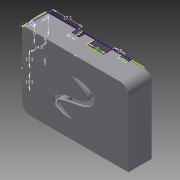
# Autodesk Inventor part: bottom
Saved by Autodesk Inventor 2015 (Build 190159000, 159)
## iProperties
Created: 2015-01-18
Part Number: bottom
Material: Generic
Document SubType Name: Modeling
Designer: Bardo91
Density: 1 g/cm^3
Appearance: Default
Author: Bardo91
Autodesk Inventor part; units mm, degrees
ref_plane "YZ Plane" through (0, 0, 0) normal (1, 0, 0) x (0, 1, 0)
ref_plane "XZ Plane" through (0, 0, 0) normal (0, 1, 0) x (-1, 0, 0)
ref_plane "XY Plane" through (0, 0, 0) normal (0, 0, 1) x (1, 0, 0)
sketch "baseBody" plane through (0, 0, 0) normal (0, 1, 0) x (-1, 0, 0)
  line L0 (50, 35) -> (-42, 35)
  line L1 (-50, 27) -> (-50, -35)
  line L2 (-50, -35) -> (42, -35)
  line L3 (50, -27) -> (50, 35)
  arc A0 (42, -35) -> (50, -27) centre (42, -27) ccw
  arc A1 (-42, 35) -> (-50, 27) centre (-42, 27) ccw
  point P0 (-50, 35)
  point P1 (50, -35)
  point P2 (0, 0)
  dimension "d175" = 100
  dimension "d176" = 70
  dimension "d177" = 50
  dimension "d178" = 35
  dimension "d179" = 8
  constraints: 8 end point, 4 point on circle, 4 point on line, 4 tangent, 2 centre point, 2 parallel, 1 equal radius, 1 horizontal, 1 perpendicular
  measures "d175" distance of point (50, -35) L1.end
  measures "d176" distance of point (-50, 35) L1.end
  measures "d177" distance from line of L1 point (0, 0)
  measures "d178" distance from line of L0 point (0, 0)
  measures "d179" radius of A0
extrude "Body" add sketch "baseBody" along normal blind 23
shell "case" thickness 2 removed faces 1 at (-16.6667, 23, 11.6667)
sketch "baseBorder" plane through (0, 23, 0) normal (0, 1, 0) x (1, 0, 0)
  line L0 (-50, -35) -> (42, -35)
  line L1 (50, -27) -> (50, 35)
  line L2 (50, 35) -> (-42, 35)
  line L3 (-50, 27) -> (-50, -35)
  arc A0 (-42, 35) -> (-50, 27) centre (-42, 27) ccw
  arc A1 (42, -35) -> (50, -27) centre (42, -27) ccw
  line L4 (42, -34) -> (-49, -34)
  line L5 (-49, -34) -> (-49, 27)
  arc A2 (-42, 34) -> (-49, 27) centre (-42, 27) ccw
  line L6 (-42, 34) -> (49, 34)
  line L7 (49, 34) -> (49, -27)
  arc A3 (42, -34) -> (49, -27) centre (42, -27) ccw
  line L8 (-48, -33) -> (42, -33)
  arc A4 (42, -33) -> (48, -27) centre (42, -27) ccw
  line L9 (48, -27) -> (48, 33)
  line L10 (48, 33) -> (-42, 33)
  arc A5 (-42, 33) -> (-48, 27) centre (-42, 27) ccw
  line L11 (-48, 27) -> (-48, -33)
  point P0 (0, 0)
  dimension "d181" = 8
  dimension "d182" = 1
  dimension "d183" = 1
  constraints: 24 end point, 12 point on circle, 6 centre point, 6 parallel, 4 tangent, 3 perpendicular, 1 equal radius, 1 horizontal, 10 other
  measures "d181" radius of A0
  measures "d182" distance between parallel lines of L0 L4
  measures "d183" distance between parallel lines of L4 L8
extrude "border" cut sketch "baseBorder" against normal blind 1 contours L3 A0 L2 L1 A1 L0
sketch "LogoSketch" plane through (0, 0, 0) normal (0, -1, 0) x (1, 0, 0)
  spline S0 degree 4 poles (-3.1163, 17.0805) (-0.2306, 16.8462) (4.559, 15.1493) (16.9576, 10.941) (13.8349, 4.9155) (11.3774, 2.8045) (7.2424, 1.6299) knots 0 0 0 0 0 0.452383 0.613098 1 1 1 1 1
  spline S1 degree 4 poles (7.2424, 1.6299) (3.9761, 0.8143) (-5.6022, -1.4455) (-10.7862, -0.979) (-21.6027, -7.4538) (-21.1895, -10.8444) (-20.3694, -14.0281) (-16.9063, -15.7155) (-14.1637, -17.0523) (-8.4251, -18.7884) (-3.6964, -18.7332) (-3.2891, -18.7749) knots 0 0 0 0 0 0.295441 0.401501 0.494293 0.5764 0.647774 0.724055 0.808389 1 1 1 1 1
  spline S2 degree 4 poles (-3.2891, -18.7749) (-6.6014, -18.3682) (-9.8767, -15.7863) (-16.2884, -14.1731) (-17.5116, -10.8025) (-17.1216, -9.3213) (-15.0626, -7.9838) (-10.1279, -6.3967) (-3.1529, -4.9614) (2.8019, -4.2581) (14.8741, -0.9961) (19.4952, 6.5686) (16.7959, 12.2137) (10.4566, 15.8501) (1.9828, 17.2619) (0.4827, 17.1476) (-3.1163, 17.0805) knots 0 0 0 0 0 0.154747 0.201512 0.240152 0.280585 0.331172 0.393993 0.472697 0.555553 0.6349 0.711183 0.78088 0.845793 1 1 1 1 1 construction
  spline S3 degree 3 poles (-2.9169, 16.547) (-0.5132, 16.1638) (4.865, 14.6593) (9.3457, 12.3941) knots 0 0 0 0 1 1 1 1
  spline S4 degree 4 poles (9.3457, 12.3941) (9.8685, 12.3683) (13.9667, 9.4075) (14.5931, 8.1931) (12.7314, 4.9035) (12.2576, 4.6291) knots 0 0 0 0 0 0.528601 1 1 1 1 1
  spline S5 degree 4 poles (-2.9169, 16.547) (-2.8752, 16.0732) (-1.741, 15.6881) (4.2878, 13.4373) (8.7044, 10.6827) (11.8989, 7.8726) (12.2576, 4.6291) knots 0 0 0 0 0 0.296538 0.478587 1 1 1 1 1
  spline S6 degree 4 poles (-3.6152, -18.2791) (-8.3434, -16.9363) (-11.1534, -14.9785) (-19.7581, -11.795) (-15.5131, -8.9995) knots 0 0 0 0 0 1 1 1 1 1
  spline S7 degree 4 poles (-3.6152, -18.2791) (-3.8818, -17.2774) (-3.4739, -17.8471) (-8.9849, -15.1901) (-10.9329, -13.7149) (-16.2763, -11.0086) (-14.5865, -8.4421) (-15.5131, -8.9995) knots 0 0 0 0 0 0.307271 0.485332 0.675667 1 1 1 1 1
  spline S8 degree 4 poles (-3.2891, -18.7749) (-6.6014, -18.3682) (-9.8767, -15.7863) (-16.2884, -14.1731) (-17.5116, -10.8025) (-17.1216, -9.3213) (-15.0626, -7.9838) (-10.1279, -6.3967) (-3.1529, -4.9614) (2.8019, -4.2581) (14.8741, -0.9961) (19.4952, 6.5686) (16.7959, 12.2137) (10.4566, 15.8501) (1.9828, 17.2619) (0.4827, 17.1476) (-3.1163, 17.0805) knots 0 0 0 0 0 0.154747 0.201512 0.240152 0.280585 0.331172 0.393993 0.472697 0.555553 0.6349 0.711183 0.78088 0.845793 1 1 1 1 1
  point P0 (0, 0)
  point P1 (1.938, 15.9498)
  point P2 (9.5194, 12.8905)
  point P3 (13.7092, 9.4987)
  point P4 (14.0418, 6.905)
  point P5 (12.5708, 4.388)
  point P6 (0, 0)
  point P7 (-8.304, -1.6299)
  point P8 (-15.513, -4.1061)
  point P9 (-20.8102, -8.4316)
  point P10 (-20.9983, -11.2525)
  point P11 (-19.8386, -13.76)
  point P12 (-17.2997, -15.5152)
  point P13 (-14.9489, -16.5809)
  point P14 (-10.5608, -17.9286)
  point P15 (-4.7622, -18.7122)
  point P16 (-8.6717, -16.9084)
  point P17 (-14.0067, -14.3212)
  point P18 (-16.7902, -12.1979)
  point P19 (-17.2997, -10.6813)
  point P20 (-17.0222, -9.6464)
  point P21 (-15.7732, -8.558)
  point P22 (-11.5623, -6.9343)
  point P23 (-4.4608, -5.3055)
  point P24 (3.0511, -3.9367)
  point P25 (14.5781, 0.8131)
  point P26 (18.0575, 7.2855)
  point P27 (11.6513, 14.727)
  point P28 (5.1387, 16.547)
  point P29 (1.0313, 17.0805)
  point P30 (16.2117, 11.7763)
  point P31 (-0.6157, 16.0547)
  point P32 (3.7776, 14.727)
  point P33 (10.9928, 11.4528)
  point P34 (13.2575, 9.2763)
  point P35 (13.7093, 7.6292)
  point P36 (13.0517, 5.6585)
  point P37 (-2.7129, 16.1985)
  point P38 (-1.5185, 15.5969)
  point P39 (2.2906, 14.0385)
  point P40 (6.6105, 11.7762)
  point P41 (10.1923, 8.8983)
  point P42 (-8.518, -16.4485)
  point P43 (-13.6523, -13.7599)
  point P44 (-16.4509, -11.1248)
  point P45 (-3.8467, -17.6058)
  point P46 (-4.4608, -17.2481)
  point P47 (-11.2887, -13.6528)
  point P48 (-14.6883, -10.6813)
  point P49 (-15.1253, -8.9995)
  point P50 (-8.304, -15.3979)
  constraints: 83 other
extrude "logo" cut sketch "LogoSketch" against normal up to next
sketch "baseFrontHoles" plane through (-50, 0, -27) normal (-1, 0, 0) x (0, 0, 1)
  line L0 (62, 0) -> (62, 10)
  line L1 (62, 0) -> (62, 22) projected
  line L2 (62, 10) -> (57.5, 10)
  line L3 (57.5, 10) -> (41.5, 10)
  line L4 (57.5, 10) -> (57.5, 23)
  line L5 (57.5, 23) -> (41.5, 23)
  line L6 (41.5, 23) -> (41.5, 10)
  line L7 (41.5, 10) -> (57.5, 10)
  line L8 (41.5, 23) -> (37.5, 23)
  line L9 (37.5, 23) -> (37.5, 8.5)
  line L10 (37.5, 8.5) -> (24, 8.5)
  line L11 (24, 8.5) -> (24, 23)
  line L12 (24, 23) -> (37.5, 23)
  line L13 (24, 23) -> (19, 23)
  line L14 (19, 23) -> (19, 8.5)
  line L15 (19, 8.5) -> (5.5, 8.5)
  line L16 (5.5, 8.5) -> (5.5, 23)
  line L17 (5.5, 23) -> (19, 23)
  point P0 (27, 0)
  dimension "d188" = 10
  dimension "d189" = 4.5
  dimension "d190" = 16
  dimension "d191" = 13
  dimension "d192" = 16
  dimension "d193" = 4
  dimension "d194" = 14.5
  dimension "d195" = 13.5
  dimension "d196" = 5
  dimension "d197" = 13.5
  constraints: 34 end point, 7 perpendicular, 6 point on line, 2 collinear, 2 horizontal, 1 vertical
  measures "d188" distance of L0.start L0.end
  measures "d189" distance of L0.end L2.end
  measures "d190" distance of L2.end L3.end
  measures "d191" distance of L2.end L4.end
  measures "d192" distance of L4.end L5.end
  measures "d193" distance of L5.end L8.end
  measures "d194" distance of L8.end L9.end
  measures "d195" distance of L9.end L10.end
  measures "d196" distance of L11.end L13.end
  measures "d197" distance of L14.end L15.end
extrude "frontHoles" cut sketch "baseFrontHoles" against normal up to surface (2 mm away)
sketch "baseLateralHoles" plane through (-50, 0, 35) normal (0, 0, 1) x (1, 0, 0)
  line L0 (2, 2) -> (2, 23)
  line L1 (2, 23) -> (29.5, 23)
  line L2 (92, 23) -> (2, 23) projected
  line L3 (29.5, 23) -> (29.5, 17)
  line L4 (29.5, 17) -> (36.5, 17)
  line L5 (36.5, 17) -> (36.5, 23)
  line L6 (29.5, 23) -> (36.5, 23)
  line L7 (36.5, 23) -> (47, 23)
  line L8 (47, 14) -> (47, 23)
  line L9 (47, 14) -> (62, 14)
  line L10 (62, 14) -> (62, 23)
  line L11 (47, 23) -> (62, 23)
  line L12 (62, 23) -> (72, 23)
  line L13 (72, 23) -> (72, 20)
  line L14 (72, 20) -> (79.5, 20)
  line L15 (79.5, 20) -> (79.5, 23)
  line L16 (72, 23) -> (79.5, 23)
  point P0 (50, 0)
  dimension "d201" = 27.5
  dimension "d202" = 6
  dimension "d203" = 7
  dimension "d204" = 15
  dimension "d205" = 10
  dimension "d206" = 7.5
  constraints: 32 end point, 9 perpendicular, 5 point on line, 3 collinear, 1 midpoint, 1 vertical
  measures "d201" distance of L0.end L1.end
  measures "d202" distance of L1.end L3.end
  measures "d203" distance of L3.end L4.end
  measures "d204" distance of L8.start L9.end
  measures "d205" distance of L10.end L12.end
  measures "d206" distance of L13.end L14.end
extrude "lateralHoles" cut sketch "baseLateralHoles" against normal up to surface (2 mm away)
ref_plane "reinforcementPlane1" through (-50, 10, 13.5) normal (0, 0, 1) x (1, 0, 0)
sketch "Sketch12" plane through (-50, 10, 13.5) normal (0, 0, 1) x (1, 0, 0)
  line L0 (2, -8) -> (2, 12)
  line L1 (8, 12) -> (1, 12) projected
  line L2 (2, 12) -> (9.0527, -8)
  line L3 (98, -8) -> (8, -8) projected
  line L4 (2, -8) -> (9.0527, -8)
  line L5 (2, -8) -> (92, -8) projected
  point P0 (50, -10)
  constraints: 6 end point, 2 point on line, 1 collinear, 1 vertical
extrude "reinforcement1" add sketch "Sketch12" against normal blind 2
ref_plane "reinforcementPlane2" through (-50, 8.5, -4) normal (0, 0, 1) x (1, 0, 0)
sketch "Sketch14" plane through (-50, 8.5, -4) normal (0, 0, 1) x (1, 0, 0)
  line L0 (9.0527, -6.5) -> (2, -6.5)
  line L1 (2, -6.5) -> (2, 13.5)
  line L2 (2, 13.5) -> (9.0527, -6.5)
  line L3 (2, 13.5) -> (9.0527, -6.5) projected
  point P0 (50, -8.5)
  constraints: 6 end point, 1 collinear, 1 horizontal, 1 perpendicular
extrude "reinforcement2" add sketch "Sketch14" against normal blind 3
ref_plane "reinforcementPlane3" through (21, 20, 35) normal (1, 0, 0) x (0, 0, -1)
sketch "Sketch15" plane through (21, 20, 35) normal (1, 0, 0) x (0, 0, -1)
  line L0 (2, -18) -> (2, 2)
  line L1 (2, 3) -> (2, -3) projected
  line L2 (2, 2) -> (9.491, -18)
  line L3 (21.5, -18) -> (2, -18) projected
  line L4 (2, -18) -> (9.491, -18)
  point P0 (35, -20)
  constraints: 6 end point, 2 point on line, 1 collinear
extrude "reinforcement3" add sketch "Sketch15" against normal blind 8
ref_plane "reinforcementPlane4" through (-4, 14, 35) normal (1, 0, 0) x (0, 0, -1)
sketch "Sketch16" plane through (-4, 14, 35) normal (1, 0, 0) x (0, 0, -1)
  line L0 (2, 8) -> (2, -12)
  line L1 (2, 8) -> (2, -12) projected
  line L2 (2, -12) -> (9.491, -12)
  line L3 (9.491, -12) -> (2, 8)
  line L4 (2, 8) -> (9.491, -12) projected
  point P0 (35, -14)
  constraints: 6 end point, 2 collinear, 1 perpendicular
extrude "reinforcement4" add sketch "Sketch16" against normal blind 8.5
sketch "Sketch17" plane through (0, 23, 0) normal (0, 1, 0) x (1, 0, 0)
  line L0 (-12.5, -33) -> (-9.5, -33)
  line L1 (-3, -33) -> (-13.5, -33) projected
  line L2 (-9.5, -33) -> (-9.5, -28)
  line L3 (-4, -33) -> (-7, -33)
  line L4 (-7, -33) -> (-7, -28)
  line L5 (-7, -28) -> (-9.5, -28)
  point P0 (0, 0)
  dimension "d223" = 3
  dimension "d224" = 5
  dimension "d225" = 3
  dimension "d226" = 5
  constraints: 10 end point, 2 perpendicular, 2 point on line
  measures "d223" distance of L0.start L0.end
  measures "d224" distance of L0.end L2.end
  measures "d225" distance of L3.start L3.end
  measures "d226" distance of L3.end L4.end
extrude "reinforcement4Hole" cut sketch "Sketch17" against normal blind 10
sketch "baseScrewHoders" plane through (-42, 2, -33) normal (0, 1, 0) x (1, 0, 0)
  line L0 (-6, -66) -> (-6, -61.6495)
  line L1 (-6, -47.5) -> (-6, -63.5) projected
  line L2 (-6, -61.6495) -> (17.575, -61.6495)
  line L3 (17.575, -61.6495) -> (17.575, -12.6995)
  line L4 (17.575, -12.6995) -> (75.075, -12.6995)
  line L5 (75.075, -12.6995) -> (75.075, -61.6495)
  line L6 (75.075, -61.6495) -> (17.575, -61.6495)
  circle A0 centre (17.575, -61.6495) radius 1.25
  circle A1 centre (17.575, -12.6995) radius 1.25
  circle A2 centre (75.075, -12.6995) radius 1.25
  circle A3 centre (75.075, -61.6495) radius 1.25
  circle A4 centre (75.075, -61.6495) radius 3
  circle A5 centre (17.575, -61.6495) radius 3
  circle A6 centre (17.575, -12.6995) radius 3
  circle A7 centre (75.075, -12.6995) radius 3
  point P0 (42, -33)
  dimension "d229" = 23.575
  dimension "d230" = 48.95
  dimension "d231" = 57.5
  dimension "d232" = 2.5
  dimension "d233" = 2.5
  dimension "d234" = 2.5
  dimension "d235" = 2.5
  dimension "d236" = 6
  dimension "d237" = 6
  dimension "d238" = 6
  dimension "d239" = 6
  dimension "d242" = 4.3505
  constraints: 12 end point, 8 centre point, 8 coincident, 4 perpendicular, 2 point on line, 1 collinear
  measures "d229" distance of L0.end L2.end
  measures "d230" distance of L2.end L3.end
  measures "d231" distance of L3.end L4.end
  measures "d232" diameter of A0
  measures "d233" diameter of A1
  measures "d234" diameter of A2
  measures "d235" diameter of A3
  measures "d236" diameter of A4
  measures "d237" diameter of A5
  measures "d238" diameter of A6
  measures "d239" diameter of A7
  measures "d242" distance of L0.start L0.end
extrude "screwHolders" add sketch "baseScrewHoders" along normal blind 16.5 contours A5 L3 A0 L2 | L2 A0 L6 A5 | A5 L6 A0 L3 | A6 L4 A1 L3 | L3 A1 L4 A6 | A4 L5 A3 L6 | L6 A3 L5 A4 | A7 L5 A2 L4 | L4 A2 L5 A7
body "Solid1"
